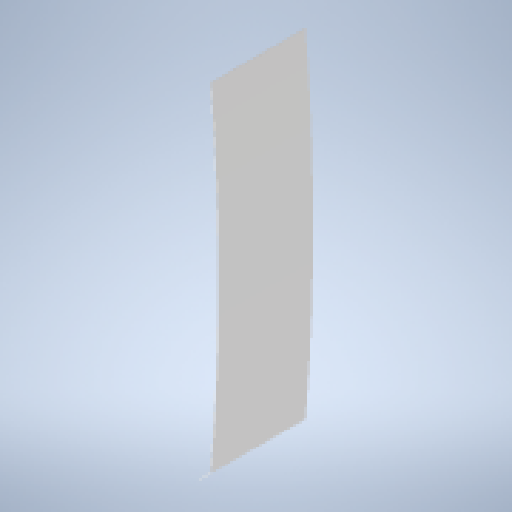
# Autodesk Inventor part: MSC 023 sheet left-right board hip
Saved by Autodesk Inventor 2025 (Build 290162010, 162A)
## iProperties
Created: 2024-04-18
Part Number: MSC 023 sheet left-right board hip
Material: Stainless Steel AISI 304
Document SubType Name: Sheet Metal
Designer: admin
Stock Number: МОО 023 лист левый-правый борт поясница
Mass: 26128.7 g
Surface Area: 21925.7 cm^2
Volume: 3266.09 cm^3
Density: 8 g/cm^3
Flat Pattern Width: 52.5 cm
Flat Pattern Length: 198.328 cm
Flat Pattern Area: 10412.2 cm^2
Sheet Metal Rule: AISI304 3mm Die 32
Sheet Metal Width: 525,000 mm
Sheet Metal Length: 1983,285 mm
Sheet Metal Area: 1041224,417 mm^2
Appearance: Default
Author: admin
Autodesk Inventor part; units mm, degrees
ref_plane "YZ Plane" through (0, 0, 0) normal (1, 0, 0) x (0, 1, 0)
ref_plane "XZ Plane" through (0, 0, 0) normal (0, 1, 0) x (-1, 0, 0)
ref_plane "XY Plane" through (0, 0, 0) normal (0, 0, 1) x (1, 0, 0)
sketch "Sketch1" plane through (0, 0, 0) normal (0, 0, 1) x (1, 0, 0)
  arc A0 (0, 0) -> (0.159434, 1.869277) centre (-11009.945504, 940) ccw construction
  arc A1 (-1.349222, -1.302929) -> (0.159434, 1.869277) centre (-4.822514, 2.29377) ccw
  line L0 (-66.367609, -75.229983) -> (-71.93398, -69.465837) construction
  line L1 (-71.93398, -69.465837) -> (-1.349222, -1.302929)
  arc A2 (0.159434, 1.869277) -> (0, 1880) centre (-11009.945504, 940) ccw
  line L2 (-1.349222, -1.302929) -> (0, 0) construction
  line L3 (0, 0) -> (0, 1880) construction
  line L4 (0, 0) -> (1.875639, 0) construction
  dimension "d148" = 5
  dimension "d153" = 100
  dimension "d165" = 11050
  dimension "d167" = 136
  dimension "d168" = 1880
  measures "d148" radius of A1
  measures "d153" distance of L2.end L1.start
  measures "d165" radius of A2
  measures "d167" angle of L2 L4
  measures "d168" distance of L2.end L3.end
contour flange "Contour Flange2" sketch "Sketch1" thickness 3 bend radius 5 width 525 along (0, 0, 1) mid plane no both sides no wall seen from (-36.641601, -35.384383, 0) lies toward (0.6946584, -0.7193398, 0) curves L1 A1 A2
bend "Bend2"
corner "Corner2"
sketch "Sketch4" plane through (-1.349222, -1.302929, 525) normal (-0.6946584, 0.7193398, 0) x (0.7193398, 0.6946584, 0)
  line L0 (-81.994451, 7.589283) -> (-81.994451, 144.595466) construction
  line L1 (-81.994451, 144.595466) -> (-67.034181, 144.595466) construction
  line L2 (-67.034181, 144.595466) -> (-67.034181, 7.589283) construction
  line L3 (-67.034181, 7.589283) -> (-81.994451, 7.589283) construction
  point P0 (1.875639, 525)
  constraints: 2 other
mark "Mark3"
equation "\"d36\" = Thickness"
equation "\"d37\" = BendReliefWidth"
equation "\"d38\" = BendReliefDepth"
equation "\"d39\" = MinimumRemnant"
equation "\"d40\" = TransitionRadius"
equation "\"d42\" = BendRadius"
equation "\"d44\" = CornerReliefSize"
equation "\"d45\" = GapSize"
equation "\"d46\" = JacobiRadiusSize"
equation "\"BendReliefWidth\" = Thickness"
equation "\"BendReliefDepth\" = 0.5 * Thickness"
equation "\"CornerReliefSize\" = 4 * Thickness"
equation "\"MinimumRemnant\" = 2 * Thickness"
equation "\"GapSize\" = Thickness"
equation "\"Thickness\" = 3"
equation "\"TransitionRadius\" = 5"
equation "\"BendRadius\" = 5"
equation "\"JacobiRadiusSize\" = 5"
body "Solid3"
